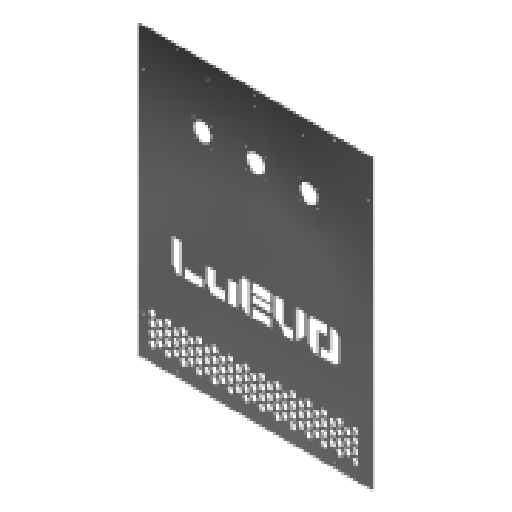
# Autodesk Inventor part: Extruder Side Panel
Saved by Autodesk Inventor 2023.2 (Build 272271000, 271)
## iProperties
Created: 2023-02-06
Part Number: Extruder Side Panel
Material: Aluminum 6061
Document SubType Name: Modeling
Designer: remop
Density: 2.7 g/cm^3
Appearance: Aluminum - Flat
Author: remop
Autodesk Inventor part; units mm, degrees
(part 1 of 2)
ref_plane "YZ Plane" through (0, 0, 0) normal (1, 0, 0) x (0, 1, 0)
ref_plane "XZ Plane" through (0, 0, 0) normal (0, 1, 0) x (-1, 0, 0)
ref_plane "XY Plane" through (0, 0, 0) normal (0, 0, 1) x (1, 0, 0)
sketch "Sketch1" plane through (0, 0, 0) normal (0, 0, 1) x (1, 0, 0)
  line L0 (-15, -15) -> (-15, 0) projected
  line L1 (0, -15) -> (-15, -15) projected
  line L2 (0, 0) -> (0, -15) projected
  line L3 (-15, 0) -> (0, 0) projected
  line L4 (360, 0) -> (360, -15) projected
  line L5 (360, -15) -> (375, -15) projected
  line L6 (375, -15) -> (375, 0) projected
  line L7 (375, 0) -> (360, 0) projected
  line L8 (360, -465) -> (360, -480) projected
  line L9 (360, -480) -> (375, -480) projected
  line L10 (375, -465) -> (375, -480) projected
  line L11 (360, -465) -> (375, -465) projected
  line L12 (0, -480) -> (0, -465) projected
  line L13 (0, -465) -> (-15, -465) projected
  line L14 (-15, -465) -> (-15, -480) projected
  line L15 (-15, -480) -> (0, -480) projected
  line L16 (375, -465) -> (375, -15)
  line L17 (360, 0) -> (0, 0)
  line L18 (-15, -15) -> (-15, -465)
  line L19 (0, -480) -> (360, -480)
  circle A0 centre (-7.5, -65) radius 1.75
  circle A1 centre (-7.5, -415) radius 1.75
  circle A2 centre (367.5, -65) radius 1.75
  circle A3 centre (367.5, -415) radius 1.75
  circle A4 centre (50, -7.5) radius 1.75
  circle A5 centre (310, -7.5) radius 1.75
  circle A6 centre (310, -472.5) radius 1.75
  circle A7 centre (50, -472.5) radius 1.75
  circle A8 centre (180, -7.5) radius 1.75
  circle A9 centre (180, -25) radius 1.75
  circle A10 centre (100, -25) radius 1.75
  circle A11 centre (260, -25) radius 1.75
  point P0 (367.5, -15)
  point P1 (367.5, -465)
  point P2 (-7.5, -465)
  point P3 (-7.5, -15)
  point P4 (0, -472.5)
  point P5 (360, -472.5)
  point P6 (0, -7.5)
  point P7 (360, -7.5)
  point P8 (180, -480)
  dimension "d0" = 50
  dimension "d1" = 3.5
  dimension "d2" = 50
  dimension "d3" = 50
  dimension "d4" = 50
  dimension "d5" = 50
  dimension "d6" = 50
  dimension "d68" = 17.5
  dimension "d69" = 80
  dimension "d70" = 80
  constraints: 12 centre point, 11 equal radius, 9 horizontal alignment, 9 midpoint, 8 end point, 6 vertical alignment, 2 perpendicular, 1 parallel, 1 vertical
  measures "d0" distance from line of A0.centre L1
  measures "d1" diameter of A2
  measures "d2" distance from line of L13 A1.centre
  measures "d3" distance from line of L12 A7.centre
  measures "d4" distance from line of A6.centre L8
  measures "d5" distance from line of L4 A5.centre
  measures "d6" distance from line of L2 A4.centre
  measures "d68" distance of A9.centre A8.centre
  measures "d69" distance of A9.centre A10.centre
  measures "d70" distance of A9.centre A11.centre
extrude "Extrusion1" add sketch "Sketch1" along normal blind 2
sketch "Sketch2" plane through (0, 0, 2) normal (0, 0, 1) x (1, 0, 0)
  line L0 (-15, -480) -> (375, -480) projected
  line L1 (375, -480) -> (375, 0) projected
  line L2 (375, 0) -> (-15, 0) projected
  line L3 (-15, 0) -> (-15, -480) projected
  circle A0 centre (50, -472.5) radius 1.75 projected
  circle A1 centre (310, -472.5) radius 1.75 projected
  circle A2 centre (310, -7.5) radius 1.75 projected
  circle A3 centre (50, -7.5) radius 1.75 projected
  circle A4 centre (367.5, -415) radius 1.75 projected
  circle A5 centre (367.5, -65) radius 1.75 projected
  circle A6 centre (-7.5, -415) radius 1.75 projected
  circle A7 centre (-7.5, -65) radius 1.75 projected
  point P0 (0, 0)
  point P1 (283.5, -90)
  point P2 (252.5, -90)
  point P3 (283.5, -121)
  point P4 (252.5, -121)
  point P5 (195.5, -90)
  point P6 (164.5, -90)
  point P7 (164.5, -121)
  point P8 (195.5, -121)
  point P9 (107.5, -90)
  point P10 (76.5, -90)
  point P11 (76.5, -121)
  point P12 (107.5, -121)
  point P13 (180, 0)
  dimension "d11" = 31
  dimension "d14" = 31
  dimension "d19" = 88
  dimension "d24" = 90
  dimension "d25" = 15.5
  constraints: 2 horizontal, 1 midpoint, 1 vertical, 11 other
  measures "d11" distance of point (283.5, -90) point (252.5, -90)
  measures "d14" distance of point (283.5, -90) point (283.5, -121)
  measures "d19" distance of point (283.5, -90) point (195.5, -90)
  measures "d24" distance from line of L2 point (76.5, -90)
  measures "d25" horizontal distance of point (180, 0) point (195.5, -90)
hole "Extruder Mount" at (283.5, -90, 2) at (252.5, -90, 2) at (283.5, -121, 2) at (252.5, -121, 2) at (195.5, -90, 2) at (164.5, -90, 2) at (164.5, -121, 2) at (195.5, -121, 2) at (107.5, -90, 2) at (76.5, -90, 2) at (76.5, -121, 2) at (107.5, -121, 2) direction (0, 0, -1) diameter 3.5 end through all
sketch "Sketch3" plane through (0, 0, 2) normal (0, 0, 1) x (1, 0, 0)
  circle A0 centre (92, -105.5) radius 15
  circle A1 centre (180, -105.5) radius 15
  circle A2 centre (268, -105.5) radius 15
  line L0 (375, 0) -> (-15, 0) projected
  point P0 (0, 0)
  point P1 (180, 0)
  dimension "d33" = 105.5
  dimension "d34" = 30
  dimension "d35" = 88
  dimension "d36" = 88
  constraints: 3 centre point, 2 equal radius, 2 horizontal alignment, 1 midpoint, 1 vertical alignment
  measures "d33" distance from line of L0 A1.centre
  measures "d34" diameter of A1
  measures "d35" distance of A1.centre A2.centre
  measures "d36" distance of A1.centre A0.centre
extrude "Extrusion2" cut sketch "Sketch3" against normal through all
sketch "Sketch4" plane through (0, 0, 2) normal (0, 0, 1) x (1, 0, 0)
  circle A0 centre (268, -105.5) radius 15 projected
  circle A1 centre (180, -105.5) radius 15 projected
  circle A2 centre (92, -105.5) radius 15 projected
  circle A3 centre (76.5, -121) radius 1.75 projected
  circle A4 centre (107.5, -90) radius 1.75 projected
  circle A5 centre (164.5, -121) radius 1.75 projected
  circle A6 centre (195.5, -90) radius 1.75 projected
  circle A7 centre (283.5, -121) radius 1.75 projected
  circle A8 centre (283.5, -90) radius 1.75 projected
  circle A9 centre (252.5, -90) radius 1.75 projected
  circle A10 centre (252.5, -121) radius 1.75 projected
  circle A11 centre (164.5, -90) radius 1.75 projected
  circle A12 centre (195.5, -121) radius 1.75 projected
  circle A13 centre (76.5, -90) radius 1.75 projected
  circle A14 centre (107.5, -121) radius 1.75 projected
  line L0 (-15, -480) -> (375, -480) projected
  line L1 (375, -480) -> (375, 0) projected
  line L2 (375, 0) -> (-15, 0) projected
  line L3 (-15, 0) -> (-15, -480) projected
  circle A15 centre (50, -472.5) radius 1.75 projected
  circle A16 centre (310, -472.5) radius 1.75 projected
  circle A17 centre (310, -7.5) radius 1.75 projected
  circle A18 centre (50, -7.5) radius 1.75 projected
  circle A19 centre (367.5, -415) radius 1.75 projected
  circle A20 centre (367.5, -65) radius 1.75 projected
  circle A21 centre (-7.5, -415) radius 1.75 projected
  circle A22 centre (-7.5, -65) radius 1.75 projected
  line L4 (10.9983, -458) -> (5.2247, -458)
  line L5 (5.2247, -458) -> (2.338, -453)
  line L6 (2.338, -453) -> (5.2247, -448)
  line L7 (5.2247, -448) -> (10.9983, -448)
  line L8 (10.9983, -448) -> (13.885, -453)
  line L9 (13.885, -453) -> (10.9983, -458)
  line L10 (18.2151, -450.5) -> (15.3284, -445.5)
  line L11 (15.3284, -445.5) -> (18.2151, -440.5)
  line L12 (18.2151, -440.5) -> (23.9886, -440.5)
  line L13 (23.9886, -440.5) -> (26.8754, -445.5)
  line L14 (26.8754, -445.5) -> (23.9886, -450.5)
  line L15 (23.9886, -450.5) -> (18.2151, -450.5)
  line L16 (10.9983, -443) -> (5.2247, -443)
  line L17 (5.2247, -443) -> (2.338, -438)
  line L18 (2.338, -438) -> (5.2247, -433)
  line L19 (5.2247, -433) -> (10.9983, -433)
  line L20 (10.9983, -433) -> (13.885, -438)
  line L21 (13.885, -438) -> (10.9983, -443)
  line L22 (5.2247, -418) -> (10.9983, -418)
  line L23 (2.338, -423) -> (5.2247, -418)
  line L24 (10.9983, -418) -> (13.885, -423)
  line L25 (18.2151, -425.5) -> (23.9886, -425.5)
  line L26 (5.2247, -428) -> (2.338, -423)
  line L27 (10.9983, -428) -> (5.2247, -428)
  line L28 (13.885, -423) -> (10.9983, -428)
  line L29 (15.3284, -430.5) -> (18.2151, -425.5)
  line L30 (23.9886, -425.5) -> (26.8754, -430.5)
  line L31 (18.2151, -435.5) -> (15.3284, -430.5)
  line L32 (23.9886, -435.5) -> (18.2151, -435.5)
  line L33 (26.8754, -430.5) -> (23.9886, -435.5)
  line L34 (5.2247, -403) -> (10.9983, -403)
  line L35 (2.338, -408) -> (5.2247, -403)
  line L36 (10.9983, -403) -> (13.885, -408)
  line L37 (18.2151, -410.5) -> (23.9886, -410.5)
  line L38 (5.2247, -413) -> (2.338, -408)
  line L39 (10.9983, -413) -> (5.2247, -413)
  line L40 (13.885, -408) -> (10.9983, -413)
  line L41 (15.3284, -415.5) -> (18.2151, -410.5)
  line L42 (23.9886, -410.5) -> (26.8754, -415.5)
  line L43 (18.2151, -420.5) -> (15.3284, -415.5)
  line L44 (23.9886, -420.5) -> (18.2151, -420.5)
  line L45 (26.8754, -415.5) -> (23.9886, -420.5)
  line L46 (36.9983, -403) -> (39.885, -408)
  line L47 (31.2247, -403) -> (36.9983, -403)
  line L48 (39.885, -408) -> (36.9983, -413)
  line L49 (28.338, -408) -> (31.2247, -403)
  line L50 (31.2247, -413) -> (28.338, -408)
  line L51 (36.9983, -413) -> (31.2247, -413)
  line L52 (44.2151, -450.5) -> (41.3284, -445.5)
  line L53 (41.3284, -445.5) -> (44.2151, -440.5)
  line L54 (44.2151, -440.5) -> (49.9886, -440.5)
  line L55 (49.9886, -440.5) -> (52.8754, -445.5)
  line L56 (49.9886, -450.5) -> (44.2151, -450.5)
  line L57 (52.8754, -445.5) -> (49.9886, -450.5)
  line L58 (36.9983, -458) -> (31.2247, -458)
  line L59 (36.9983, -448) -> (39.885, -453)
  line L60 (39.885, -438) -> (36.9983, -443)
  line L61 (39.885, -453) -> (36.9983, -458)
  line L62 (31.2247, -448) -> (36.9983, -448)
  line L63 (31.2247, -458) -> (28.338, -453)
  line L64 (28.338, -453) -> (31.2247, -448)
  line L65 (36.9983, -433) -> (39.885, -438)
  line L66 (36.9983, -443) -> (31.2247, -443)
  line L67 (31.2247, -443) -> (28.338, -438)
  line L68 (31.2247, -433) -> (36.9983, -433)
  line L69 (28.338, -438) -> (31.2247, -433)
  line L70 (36.9983, -428) -> (31.2247, -428)
  line L71 (39.885, -423) -> (36.9983, -428)
  line L72 (31.2247, -428) -> (28.338, -423)
  line L73 (36.9983, -418) -> (39.885, -423)
  line L74 (31.2247, -418) -> (36.9983, -418)
  line L75 (28.338, -423) -> (31.2247, -418)
  line L76 (41.3284, -430.5) -> (44.2151, -425.5)
  line L77 (44.2151, -435.5) -> (41.3284, -430.5)
  line L78 (49.9886, -435.5) -> (44.2151, -435.5)
  line L79 (52.8754, -430.5) -> (49.9886, -435.5)
  line L80 (49.9886, -425.5) -> (52.8754, -430.5)
  line L81 (44.2151, -425.5) -> (49.9886, -425.5)
  line L82 (44.2151, -420.5) -> (41.3284, -415.5)
  line L83 (41.3284, -415.5) -> (44.2151, -410.5)
  line L84 (49.9886, -420.5) -> (44.2151, -420.5)
  line L85 (44.2151, -410.5) -> (49.9886, -410.5)
  line L86 (52.8754, -415.5) -> (49.9886, -420.5)
  line L87 (49.9886, -410.5) -> (52.8754, -415.5)
  line L88 (62.9983, -403) -> (65.885, -408)
  line L89 (57.2247, -403) -> (62.9983, -403)
  line L90 (65.885, -408) -> (62.9983, -413)
  line L91 (54.338, -408) -> (57.2247, -403)
  line L92 (57.2247, -413) -> (54.338, -408)
  line L93 (62.9983, -413) -> (57.2247, -413)
  line L94 (70.2151, -450.5) -> (67.3284, -445.5)
  line L95 (67.3284, -445.5) -> (70.2151, -440.5)
  line L96 (70.2151, -440.5) -> (75.9886, -440.5)
  line L97 (75.9886, -440.5) -> (78.8754, -445.5)
  line L98 (75.9886, -450.5) -> (70.2151, -450.5)
  line L99 (78.8754, -445.5) -> (75.9886, -450.5)
  line L100 (62.9983, -458) -> (57.2247, -458)
  line L101 (62.9983, -448) -> (65.885, -453)
  line L102 (65.885, -438) -> (62.9983, -443)
  line L103 (65.885, -453) -> (62.9983, -458)
  line L104 (57.2247, -448) -> (62.9983, -448)
  line L105 (57.2247, -458) -> (54.338, -453)
  line L106 (54.338, -453) -> (57.2247, -448)
  line L107 (62.9983, -433) -> (65.885, -438)
  line L108 (62.9983, -443) -> (57.2247, -443)
  line L109 (57.2247, -443) -> (54.338, -438)
  line L110 (57.2247, -433) -> (62.9983, -433)
  line L111 (54.338, -438) -> (57.2247, -433)
  line L112 (62.9983, -428) -> (57.2247, -428)
  line L113 (65.885, -423) -> (62.9983, -428)
  line L114 (57.2247, -428) -> (54.338, -423)
  line L115 (62.9983, -418) -> (65.885, -423)
  line L116 (57.2247, -418) -> (62.9983, -418)
  line L117 (54.338, -423) -> (57.2247, -418)
  line L118 (67.3284, -430.5) -> (70.2151, -425.5)
  line L119 (70.2151, -435.5) -> (67.3284, -430.5)
  line L120 (75.9886, -435.5) -> (70.2151, -435.5)
  line L121 (78.8754, -430.5) -> (75.9886, -435.5)
  line L122 (75.9886, -425.5) -> (78.8754, -430.5)
  line L123 (70.2151, -425.5) -> (75.9886, -425.5)
  line L124 (70.2151, -420.5) -> (67.3284, -415.5)
  line L125 (67.3284, -415.5) -> (70.2151, -410.5)
  line L126 (75.9886, -420.5) -> (70.2151, -420.5)
  line L127 (70.2151, -410.5) -> (75.9886, -410.5)
  line L128 (78.8754, -415.5) -> (75.9886, -420.5)
  line L129 (75.9886, -410.5) -> (78.8754, -415.5)
  line L130 (88.9983, -403) -> (91.885, -408)
  line L131 (83.2247, -403) -> (88.9983, -403)
  line L132 (91.885, -408) -> (88.9983, -413)
  line L133 (80.338, -408) -> (83.2247, -403)
  line L134 (83.2247, -413) -> (80.338, -408)
  line L135 (88.9983, -413) -> (83.2247, -413)
  line L136 (96.2151, -450.5) -> (93.3284, -445.5)
  line L137 (93.3284, -445.5) -> (96.2151, -440.5)
  line L138 (96.2151, -440.5) -> (101.9886, -440.5)
  line L139 (101.9886, -440.5) -> (104.8754, -445.5)
  line L140 (101.9886, -450.5) -> (96.2151, -450.5)
  line L141 (104.8754, -445.5) -> (101.9886, -450.5)
  line L142 (88.9983, -458) -> (83.2247, -458)
  line L143 (88.9983, -448) -> (91.885, -453)
  line L144 (91.885, -438) -> (88.9983, -443)
  line L145 (91.885, -453) -> (88.9983, -458)
  line L146 (83.2247, -448) -> (88.9983, -448)
  line L147 (83.2247, -458) -> (80.338, -453)
  line L148 (80.338, -453) -> (83.2247, -448)
  line L149 (88.9983, -433) -> (91.885, -438)
  line L150 (88.9983, -443) -> (83.2247, -443)
  line L151 (83.2247, -443) -> (80.338, -438)
  line L152 (83.2247, -433) -> (88.9983, -433)
  line L153 (80.338, -438) -> (83.2247, -433)
  line L154 (88.9983, -428) -> (83.2247, -428)
  line L155 (91.885, -423) -> (88.9983, -428)
  line L156 (83.2247, -428) -> (80.338, -423)
  line L157 (88.9983, -418) -> (91.885, -423)
  line L158 (83.2247, -418) -> (88.9983, -418)
  line L159 (80.338, -423) -> (83.2247, -418)
  line L160 (93.3284, -430.5) -> (96.2151, -425.5)
  line L161 (96.2151, -435.5) -> (93.3284, -430.5)
  line L162 (101.9886, -435.5) -> (96.2151, -435.5)
  line L163 (104.8754, -430.5) -> (101.9886, -435.5)
  line L164 (101.9886, -425.5) -> (104.8754, -430.5)
  line L165 (96.2151, -425.5) -> (101.9886, -425.5)
  line L166 (96.2151, -420.5) -> (93.3284, -415.5)
  line L167 (93.3284, -415.5) -> (96.2151, -410.5)
  line L168 (101.9886, -420.5) -> (96.2151, -420.5)
  line L169 (96.2151, -410.5) -> (101.9886, -410.5)
  line L170 (104.8754, -415.5) -> (101.9886, -420.5)
  line L171 (101.9886, -410.5) -> (104.8754, -415.5)
  line L172 (114.9983, -403) -> (117.885, -408)
  line L173 (109.2247, -403) -> (114.9983, -403)
  line L174 (117.885, -408) -> (114.9983, -413)
  line L175 (106.338, -408) -> (109.2247, -403)
  line L176 (109.2247, -413) -> (106.338, -408)
  line L177 (114.9983, -413) -> (109.2247, -413)
  line L178 (122.2151, -450.5) -> (119.3284, -445.5)
  line L179 (119.3284, -445.5) -> (122.2151, -440.5)
  line L180 (122.2151, -440.5) -> (127.9886, -440.5)
  line L181 (127.9886, -440.5) -> (130.8754, -445.5)
  line L182 (127.9886, -450.5) -> (122.2151, -450.5)
  line L183 (130.8754, -445.5) -> (127.9886, -450.5)
  line L184 (114.9983, -458) -> (109.2247, -458)
  line L185 (114.9983, -448) -> (117.885, -453)
  line L186 (117.885, -438) -> (114.9983, -443)
  line L187 (117.885, -453) -> (114.9983, -458)
  line L188 (109.2247, -448) -> (114.9983, -448)
  line L189 (109.2247, -458) -> (106.338, -453)
  line L190 (106.338, -453) -> (109.2247, -448)
  line L191 (114.9983, -433) -> (117.885, -438)
  line L192 (114.9983, -443) -> (109.2247, -443)
  line L193 (109.2247, -443) -> (106.338, -438)
  line L194 (109.2247, -433) -> (114.9983, -433)
  line L195 (106.338, -438) -> (109.2247, -433)
  line L196 (114.9983, -428) -> (109.2247, -428)
  line L197 (117.885, -423) -> (114.9983, -428)
  line L198 (109.2247, -428) -> (106.338, -423)
  line L199 (114.9983, -418) -> (117.885, -423)
  line L200 (109.2247, -418) -> (114.9983, -418)
  line L201 (106.338, -423) -> (109.2247, -418)
  line L202 (119.3284, -430.5) -> (122.2151, -425.5)
  line L203 (122.2151, -435.5) -> (119.3284, -430.5)
  line L204 (127.9886, -435.5) -> (122.2151, -435.5)
  line L205 (130.8754, -430.5) -> (127.9886, -435.5)
  line L206 (127.9886, -425.5) -> (130.8754, -430.5)
  line L207 (122.2151, -425.5) -> (127.9886, -425.5)
  line L208 (122.2151, -420.5) -> (119.3284, -415.5)
  line L209 (119.3284, -415.5) -> (122.2151, -410.5)
  line L210 (127.9886, -420.5) -> (122.2151, -420.5)
  line L211 (122.2151, -410.5) -> (127.9886, -410.5)
  line L212 (130.8754, -415.5) -> (127.9886, -420.5)
  line L213 (127.9886, -410.5) -> (130.8754, -415.5)
  line L214 (140.9983, -403) -> (143.885, -408)
  line L215 (135.2247, -403) -> (140.9983, -403)
  line L216 (143.885, -408) -> (140.9983, -413)
  line L217 (132.338, -408) -> (135.2247, -403)
  line L218 (135.2247, -413) -> (132.338, -408)
  line L219 (140.9983, -413) -> (135.2247, -413)
  line L220 (148.2151, -450.5) -> (145.3284, -445.5)
  line L221 (145.3284, -445.5) -> (148.2151, -440.5)
  line L222 (148.2151, -440.5) -> (153.9886, -440.5)
  line L223 (153.9886, -440.5) -> (156.8754, -445.5)
  line L224 (153.9886, -450.5) -> (148.2151, -450.5)
  line L225 (156.8754, -445.5) -> (153.9886, -450.5)
  line L226 (140.9983, -458) -> (135.2247, -458)
  line L227 (140.9983, -448) -> (143.885, -453)
  line L228 (143.885, -438) -> (140.9983, -443)
  line L229 (143.885, -453) -> (140.9983, -458)
  line L230 (135.2247, -448) -> (140.9983, -448)
  line L231 (135.2247, -458) -> (132.338, -453)
  line L232 (132.338, -453) -> (135.2247, -448)
  line L233 (140.9983, -433) -> (143.885, -438)
  line L234 (140.9983, -443) -> (135.2247, -443)
  line L235 (135.2247, -443) -> (132.338, -438)
  line L236 (135.2247, -433) -> (140.9983, -433)
  line L237 (132.338, -438) -> (135.2247, -433)
  line L238 (140.9983, -428) -> (135.2247, -428)
  line L239 (143.885, -423) -> (140.9983, -428)
  line L240 (135.2247, -428) -> (132.338, -423)
  line L241 (140.9983, -418) -> (143.885, -423)
  line L242 (135.2247, -418) -> (140.9983, -418)
  line L243 (132.338, -423) -> (135.2247, -418)
  line L244 (145.3284, -430.5) -> (148.2151, -425.5)
  line L245 (148.2151, -435.5) -> (145.3284, -430.5)
  line L246 (153.9886, -435.5) -> (148.2151, -435.5)
  line L247 (156.8754, -430.5) -> (153.9886, -435.5)
  line L248 (153.9886, -425.5) -> (156.8754, -430.5)
  line L249 (148.2151, -425.5) -> (153.9886, -425.5)
  line L250 (148.2151, -420.5) -> (145.3284, -415.5)
  line L251 (145.3284, -415.5) -> (148.2151, -410.5)
  line L252 (153.9886, -420.5) -> (148.2151, -420.5)
  line L253 (148.2151, -410.5) -> (153.9886, -410.5)
  line L254 (156.8754, -415.5) -> (153.9886, -420.5)
  line L255 (153.9886, -410.5) -> (156.8754, -415.5)
  line L256 (166.9983, -403) -> (169.885, -408)
  line L257 (161.2247, -403) -> (166.9983, -403)
  line L258 (169.885, -408) -> (166.9983, -413)
  line L259 (158.338, -408) -> (161.2247, -403)
  line L260 (161.2247, -413) -> (158.338, -408)
  line L261 (166.9983, -413) -> (161.2247, -413)
  line L262 (174.2151, -450.5) -> (171.3284, -445.5)
  line L263 (171.3284, -445.5) -> (174.2151, -440.5)
  line L264 (174.2151, -440.5) -> (179.9886, -440.5)
  line L265 (179.9886, -440.5) -> (182.8754, -445.5)
  line L266 (179.9886, -450.5) -> (174.2151, -450.5)
  line L267 (182.8754, -445.5) -> (179.9886, -450.5)
  line L268 (166.9983, -458) -> (161.2247, -458)
  line L269 (166.9983, -448) -> (169.885, -453)
  line L270 (169.885, -438) -> (166.9983, -443)
  line L271 (169.885, -453) -> (166.9983, -458)
  line L272 (161.2247, -448) -> (166.9983, -448)
  line L273 (161.2247, -458) -> (158.338, -453)
  line L274 (158.338, -453) -> (161.2247, -448)
  line L275 (166.9983, -433) -> (169.885, -438)
  line L276 (166.9983, -443) -> (161.2247, -443)
  line L277 (161.2247, -443) -> (158.338, -438)
  line L278 (161.2247, -433) -> (166.9983, -433)
  line L279 (158.338, -438) -> (161.2247, -433)
  line L280 (166.9983, -428) -> (161.2247, -428)
  line L281 (169.885, -423) -> (166.9983, -428)
  line L282 (161.2247, -428) -> (158.338, -423)
  line L283 (166.9983, -418) -> (169.885, -423)
  line L284 (161.2247, -418) -> (166.9983, -418)
  line L285 (158.338, -423) -> (161.2247, -418)
  line L286 (171.3284, -430.5) -> (174.2151, -425.5)
  line L287 (174.2151, -435.5) -> (171.3284, -430.5)
  line L288 (179.9886, -435.5) -> (174.2151, -435.5)
  line L289 (182.8754, -430.5) -> (179.9886, -435.5)
  line L290 (179.9886, -425.5) -> (182.8754, -430.5)
  line L291 (174.2151, -425.5) -> (179.9886, -425.5)
  line L292 (174.2151, -420.5) -> (171.3284, -415.5)
  line L293 (171.3284, -415.5) -> (174.2151, -410.5)
  line L294 (179.9886, -420.5) -> (174.2151, -420.5)
  line L295 (174.2151, -410.5) -> (179.9886, -410.5)
  line L296 (182.8754, -415.5) -> (179.9886, -420.5)
  line L297 (179.9886, -410.5) -> (182.8754, -415.5)
  line L298 (192.9983, -403) -> (195.885, -408)
  line L299 (187.2247, -403) -> (192.9983, -403)
  line L300 (195.885, -408) -> (192.9983, -413)
  line L301 (184.338, -408) -> (187.2247, -403)
  line L302 (187.2247, -413) -> (184.338, -408)
  line L303 (192.9983, -413) -> (187.2247, -413)
  line L304 (200.2151, -450.5) -> (197.3284, -445.5)
  line L305 (197.3284, -445.5) -> (200.2151, -440.5)
  line L306 (200.2151, -440.5) -> (205.9886, -440.5)
  line L307 (205.9886, -440.5) -> (208.8754, -445.5)
  line L308 (205.9886, -450.5) -> (200.2151, -450.5)
  line L309 (208.8754, -445.5) -> (205.9886, -450.5)
  line L310 (192.9983, -458) -> (187.2247, -458)
  line L311 (192.9983, -448) -> (195.885, -453)
  line L312 (195.885, -438) -> (192.9983, -443)
  line L313 (195.885, -453) -> (192.9983, -458)
  line L314 (187.2247, -448) -> (192.9983, -448)
  line L315 (187.2247, -458) -> (184.338, -453)
  line L316 (184.338, -453) -> (187.2247, -448)
  line L317 (192.9983, -433) -> (195.885, -438)
  line L318 (192.9983, -443) -> (187.2247, -443)
  line L319 (187.2247, -443) -> (184.338, -438)
  line L320 (187.2247, -433) -> (192.9983, -433)
  line L321 (184.338, -438) -> (187.2247, -433)
  line L322 (192.9983, -428) -> (187.2247, -428)
  line L323 (195.885, -423) -> (192.9983, -428)
  line L324 (187.2247, -428) -> (184.338, -423)
  line L325 (192.9983, -418) -> (195.885, -423)
  line L326 (187.2247, -418) -> (192.9983, -418)
  line L327 (184.338, -423) -> (187.2247, -418)
  line L328 (197.3284, -430.5) -> (200.2151, -425.5)
  line L329 (200.2151, -435.5) -> (197.3284, -430.5)
  line L330 (205.9886, -435.5) -> (200.2151, -435.5)
  line L331 (208.8754, -430.5) -> (205.9886, -435.5)
  line L332 (205.9886, -425.5) -> (208.8754, -430.5)
  line L333 (200.2151, -425.5) -> (205.9886, -425.5)
  line L334 (200.2151, -420.5) -> (197.3284, -415.5)
  line L335 (197.3284, -415.5) -> (200.2151, -410.5)
  line L336 (205.9886, -420.5) -> (200.2151, -420.5)
  line L337 (200.2151, -410.5) -> (205.9886, -410.5)
  line L338 (208.8754, -415.5) -> (205.9886, -420.5)
  line L339 (205.9886, -410.5) -> (208.8754, -415.5)
  line L340 (218.9983, -403) -> (221.885, -408)
  line L341 (213.2247, -403) -> (218.9983, -403)
  line L342 (221.885, -408) -> (218.9983, -413)
  line L343 (210.338, -408) -> (213.2247, -403)
  line L344 (213.2247, -413) -> (210.338, -408)
  line L345 (218.9983, -413) -> (213.2247, -413)
  line L346 (226.2151, -450.5) -> (223.3284, -445.5)
  line L347 (223.3284, -445.5) -> (226.2151, -440.5)
  line L348 (226.2151, -440.5) -> (231.9886, -440.5)
  line L349 (231.9886, -440.5) -> (234.8754, -445.5)
  line L350 (231.9886, -450.5) -> (226.2151, -450.5)
  line L351 (234.8754, -445.5) -> (231.9886, -450.5)
  line L352 (218.9983, -458) -> (213.2247, -458)
  line L353 (218.9983, -448) -> (221.885, -453)
  line L354 (221.885, -438) -> (218.9983, -443)
  line L355 (221.885, -453) -> (218.9983, -458)
  line L356 (213.2247, -448) -> (218.9983, -448)
  line L357 (213.2247, -458) -> (210.338, -453)
  line L358 (210.338, -453) -> (213.2247, -448)
  line L359 (218.9983, -433) -> (221.885, -438)
  line L360 (218.9983, -443) -> (213.2247, -443)
  line L361 (213.2247, -443) -> (210.338, -438)
  line L362 (213.2247, -433) -> (218.9983, -433)
  line L363 (210.338, -438) -> (213.2247, -433)
  line L364 (218.9983, -428) -> (213.2247, -428)
  line L365 (221.885, -423) -> (218.9983, -428)
  line L366 (213.2247, -428) -> (210.338, -423)
  line L367 (218.9983, -418) -> (221.885, -423)
  line L368 (213.2247, -418) -> (218.9983, -418)
  line L369 (210.338, -423) -> (213.2247, -418)
  line L370 (223.3284, -430.5) -> (226.2151, -425.5)
  line L371 (226.2151, -435.5) -> (223.3284, -430.5)
  line L372 (231.9886, -435.5) -> (226.2151, -435.5)
  line L373 (234.8754, -430.5) -> (231.9886, -435.5)
  line L374 (231.9886, -425.5) -> (234.8754, -430.5)
  line L375 (226.2151, -425.5) -> (231.9886, -425.5)
  line L376 (226.2151, -420.5) -> (223.3284, -415.5)
  line L377 (223.3284, -415.5) -> (226.2151, -410.5)
  line L378 (231.9886, -420.5) -> (226.2151, -420.5)
  line L379 (226.2151, -410.5) -> (231.9886, -410.5)
  line L380 (234.8754, -415.5) -> (231.9886, -420.5)
  line L381 (231.9886, -410.5) -> (234.8754, -415.5)
  line L382 (244.9983, -403) -> (247.885, -408)
  line L383 (239.2247, -403) -> (244.9983, -403)
  line L384 (247.885, -408) -> (244.9983, -413)
  line L385 (236.338, -408) -> (239.2247, -403)
  line L386 (239.2247, -413) -> (236.338, -408)
  line L387 (244.9983, -413) -> (239.2247, -413)
  line L388 (252.2151, -450.5) -> (249.3284, -445.5)
  line L389 (249.3284, -445.5) -> (252.2151, -440.5)
  line L390 (252.2151, -440.5) -> (257.9886, -440.5)
  line L391 (257.9886, -440.5) -> (260.8754, -445.5)
  line L392 (257.9886, -450.5) -> (252.2151, -450.5)
  line L393 (260.8754, -445.5) -> (257.9886, -450.5)
  line L394 (244.9983, -458) -> (239.2247, -458)
  line L395 (244.9983, -448) -> (247.885, -453)
  line L396 (247.885, -438) -> (244.9983, -443)
  line L397 (247.885, -453) -> (244.9983, -458)
  line L398 (239.2247, -448) -> (244.9983, -448)
  line L399 (239.2247, -458) -> (236.338, -453)
  line L400 (236.338, -453) -> (239.2247, -448)
  line L401 (244.9983, -433) -> (247.885, -438)
  line L402 (244.9983, -443) -> (239.2247, -443)
  line L403 (239.2247, -443) -> (236.338, -438)
  line L404 (239.2247, -433) -> (244.9983, -433)
  line L405 (236.338, -438) -> (239.2247, -433)
  line L406 (244.9983, -428) -> (239.2247, -428)
  line L407 (247.885, -423) -> (244.9983, -428)
  line L408 (239.2247, -428) -> (236.338, -423)
  line L409 (244.9983, -418) -> (247.885, -423)
  line L410 (239.2247, -418) -> (244.9983, -418)
  line L411 (236.338, -423) -> (239.2247, -418)
  line L412 (249.3284, -430.5) -> (252.2151, -425.5)
  line L413 (252.2151, -435.5) -> (249.3284, -430.5)
  line L414 (257.9886, -435.5) -> (252.2151, -435.5)
  line L415 (260.8754, -430.5) -> (257.9886, -435.5)
  line L416 (257.9886, -425.5) -> (260.8754, -430.5)
  line L417 (252.2151, -425.5) -> (257.9886, -425.5)
  line L418 (252.2151, -420.5) -> (249.3284, -415.5)
  line L419 (249.3284, -415.5) -> (252.2151, -410.5)
  line L420 (257.9886, -420.5) -> (252.2151, -420.5)
  line L421 (252.2151, -410.5) -> (257.9886, -410.5)
  line L422 (260.8754, -415.5) -> (257.9886, -420.5)
  line L423 (257.9886, -410.5) -> (260.8754, -415.5)
  line L424 (270.9983, -403) -> (273.885, -408)
  line L425 (265.2247, -403) -> (270.9983, -403)
  line L426 (273.885, -408) -> (270.9983, -413)
  line L427 (262.338, -408) -> (265.2247, -403)
  line L428 (265.2247, -413) -> (262.338, -408)
  line L429 (270.9983, -413) -> (265.2247, -413)
  line L430 (278.2151, -450.5) -> (275.3284, -445.5)
  line L431 (275.3284, -445.5) -> (278.2151, -440.5)
  line L432 (278.2151, -440.5) -> (283.9886, -440.5)
  line L433 (283.9886, -440.5) -> (286.8754, -445.5)
  line L434 (283.9886, -450.5) -> (278.2151, -450.5)
  line L435 (286.8754, -445.5) -> (283.9886, -450.5)
  line L436 (270.9983, -458) -> (265.2247, -458)
  line L437 (270.9983, -448) -> (273.885, -453)
  line L438 (273.885, -438) -> (270.9983, -443)
  line L439 (273.885, -453) -> (270.9983, -458)
  line L440 (265.2247, -448) -> (270.9983, -448)
  line L441 (265.2247, -458) -> (262.338, -453)
  line L442 (262.338, -453) -> (265.2247, -448)
  line L443 (270.9983, -433) -> (273.885, -438)
  line L444 (270.9983, -443) -> (265.2247, -443)
  line L445 (265.2247, -443) -> (262.338, -438)
  line L446 (265.2247, -433) -> (270.9983, -433)
  line L447 (262.338, -438) -> (265.2247, -433)
  line L448 (270.9983, -428) -> (265.2247, -428)
  line L449 (273.885, -423) -> (270.9983, -428)
  line L450 (265.2247, -428) -> (262.338, -423)
  line L451 (270.9983, -418) -> (273.885, -423)
  line L452 (265.2247, -418) -> (270.9983, -418)
  line L453 (262.338, -423) -> (265.2247, -418)
  line L454 (275.3284, -430.5) -> (278.2151, -425.5)
  line L455 (278.2151, -435.5) -> (275.3284, -430.5)
  line L456 (283.9886, -435.5) -> (278.2151, -435.5)
  line L457 (286.8754, -430.5) -> (283.9886, -435.5)
  line L458 (283.9886, -425.5) -> (286.8754, -430.5)
  line L459 (278.2151, -425.5) -> (283.9886, -425.5)
  line L460 (278.2151, -420.5) -> (275.3284, -415.5)
  line L461 (275.3284, -415.5) -> (278.2151, -410.5)
  line L462 (283.9886, -420.5) -> (278.2151, -420.5)
  line L463 (278.2151, -410.5) -> (283.9886, -410.5)
  line L464 (286.8754, -415.5) -> (283.9886, -420.5)
  line L465 (283.9886, -410.5) -> (286.8754, -415.5)
  line L466 (296.9983, -403) -> (299.885, -408)
  line L467 (291.2247, -403) -> (296.9983, -403)
  line L468 (299.885, -408) -> (296.9983, -413)
  line L469 (288.338, -408) -> (291.2247, -403)
  line L470 (291.2247, -413) -> (288.338, -408)
  line L471 (296.9983, -413) -> (291.2247, -413)
  line L472 (304.2151, -450.5) -> (301.3284, -445.5)
  line L473 (301.3284, -445.5) -> (304.2151, -440.5)
  line L474 (304.2151, -440.5) -> (309.9886, -440.5)
  line L475 (309.9886, -440.5) -> (312.8754, -445.5)
  line L476 (309.9886, -450.5) -> (304.2151, -450.5)
  line L477 (312.8754, -445.5) -> (309.9886, -450.5)
  line L478 (296.9983, -458) -> (291.2247, -458)
  line L479 (296.9983, -448) -> (299.885, -453)
  line L480 (299.885, -438) -> (296.9983, -443)
  line L481 (299.885, -453) -> (296.9983, -458)
  line L482 (291.2247, -448) -> (296.9983, -448)
  line L483 (291.2247, -458) -> (288.338, -453)
  line L484 (288.338, -453) -> (291.2247, -448)
  line L485 (296.9983, -433) -> (299.885, -438)
  line L486 (296.9983, -443) -> (291.2247, -443)
  line L487 (291.2247, -443) -> (288.338, -438)
  line L488 (291.2247, -433) -> (296.9983, -433)
  line L489 (288.338, -438) -> (291.2247, -433)
  line L490 (296.9983, -428) -> (291.2247, -428)
  line L491 (299.885, -423) -> (296.9983, -428)
  line L492 (291.2247, -428) -> (288.338, -423)
  line L493 (296.9983, -418) -> (299.885, -423)
  line L494 (291.2247, -418) -> (296.9983, -418)
  line L495 (288.338, -423) -> (291.2247, -418)
  line L496 (301.3284, -430.5) -> (304.2151, -425.5)
  line L497 (304.2151, -435.5) -> (301.3284, -430.5)
  line L498 (309.9886, -435.5) -> (304.2151, -435.5)
  line L499 (312.8754, -430.5) -> (309.9886, -435.5)
  line L500 (309.9886, -425.5) -> (312.8754, -430.5)
  line L501 (304.2151, -425.5) -> (309.9886, -425.5)
  line L502 (304.2151, -420.5) -> (301.3284, -415.5)
  line L503 (301.3284, -415.5) -> (304.2151, -410.5)
  line L504 (309.9886, -420.5) -> (304.2151, -420.5)
  line L505 (304.2151, -410.5) -> (309.9886, -410.5)
  line L506 (312.8754, -415.5) -> (309.9886, -420.5)
  line L507 (309.9886, -410.5) -> (312.8754, -415.5)
  line L508 (322.9983, -403) -> (325.885, -408)
  line L509 (317.2247, -403) -> (322.9983, -403)
  line L510 (325.885, -408) -> (322.9983, -413)
  line L511 (314.338, -408) -> (317.2247, -403)
  line L512 (317.2247, -413) -> (314.338, -408)
  line L513 (322.9983, -413) -> (317.2247, -413)
  line L514 (330.2151, -450.5) -> (327.3284, -445.5)
  line L515 (327.3284, -445.5) -> (330.2151, -440.5)
  line L516 (330.2151, -440.5) -> (335.9886, -440.5)
  line L517 (335.9886, -440.5) -> (338.8754, -445.5)
  line L518 (335.9886, -450.5) -> (330.2151, -450.5)
  line L519 (338.8754, -445.5) -> (335.9886, -450.5)
  line L520 (322.9983, -458) -> (317.2247, -458)
  line L521 (322.9983, -448) -> (325.885, -453)
  line L522 (325.885, -438) -> (322.9983, -443)
  line L523 (325.885, -453) -> (322.9983, -458)
  line L524 (317.2247, -448) -> (322.9983, -448)
  line L525 (317.2247, -458) -> (314.338, -453)
  line L526 (314.338, -453) -> (317.2247, -448)
  line L527 (322.9983, -433) -> (325.885, -438)
  line L528 (322.9983, -443) -> (317.2247, -443)
  line L529 (317.2247, -443) -> (314.338, -438)
  line L530 (317.2247, -433) -> (322.9983, -433)
  line L531 (314.338, -438) -> (317.2247, -433)
  line L532 (322.9983, -428) -> (317.2247, -428)
  line L533 (325.885, -423) -> (322.9983, -428)
  line L534 (317.2247, -428) -> (314.338, -423)
  line L535 (322.9983, -418) -> (325.885, -423)
  line L536 (317.2247, -418) -> (322.9983, -418)
  line L537 (314.338, -423) -> (317.2247, -418)
  line L538 (327.3284, -430.5) -> (330.2151, -425.5)
  line L539 (330.2151, -435.5) -> (327.3284, -430.5)
  line L540 (335.9886, -435.5) -> (330.2151, -435.5)
  line L541 (338.8754, -430.5) -> (335.9886, -435.5)
  line L542 (335.9886, -425.5) -> (338.8754, -430.5)
  line L543 (330.2151, -425.5) -> (335.9886, -425.5)
  line L544 (330.2151, -420.5) -> (327.3284, -415.5)
  line L545 (327.3284, -415.5) -> (330.2151, -410.5)
  line L546 (335.9886, -420.5) -> (330.2151, -420.5)
  line L547 (330.2151, -410.5) -> (335.9886, -410.5)
  line L548 (338.8754, -415.5) -> (335.9886, -420.5)
  line L549 (335.9886, -410.5) -> (338.8754, -415.5)
  line L550 (348.9983, -403) -> (351.885, -408)
  line L551 (343.2247, -403) -> (348.9983, -403)
  line L552 (351.885, -408) -> (348.9983, -413)
  line L553 (340.338, -408) -> (343.2247, -403)
  line L554 (343.2247, -413) -> (340.338, -408)
  line L555 (348.9983, -413) -> (343.2247, -413)
  line L556 (356.2151, -450.5) -> (353.3284, -445.5)
  line L557 (353.3284, -445.5) -> (356.2151, -440.5)
  line L558 (356.2151, -440.5) -> (361.9886, -440.5)
  line L559 (361.9886, -440.5) -> (364.8754, -445.5)
  line L560 (361.9886, -450.5) -> (356.2151, -450.5)
  line L561 (364.8754, -445.5) -> (361.9886, -450.5)
  line L562 (348.9983, -458) -> (343.2247, -458)
  line L563 (348.9983, -448) -> (351.885, -453)
  line L564 (351.885, -438) -> (348.9983, -443)
  line L565 (351.885, -453) -> (348.9983, -458)
  line L566 (343.2247, -448) -> (348.9983, -448)
  line L567 (343.2247, -458) -> (340.338, -453)
  line L568 (340.338, -453) -> (343.2247, -448)
  line L569 (348.9983, -433) -> (351.885, -438)
  line L570 (348.9983, -443) -> (343.2247, -443)
  line L571 (343.2247, -443) -> (340.338, -438)
  line L572 (343.2247, -433) -> (348.9983, -433)
  line L573 (340.338, -438) -> (343.2247, -433)
  line L574 (348.9983, -428) -> (343.2247, -428)
  line L575 (351.885, -423) -> (348.9983, -428)
  line L576 (343.2247, -428) -> (340.338, -423)
  line L577 (348.9983, -418) -> (351.885, -423)
  line L578 (343.2247, -418) -> (348.9983, -418)
  line L579 (340.338, -423) -> (343.2247, -418)
  line L580 (353.3284, -430.5) -> (356.2151, -425.5)
  line L581 (356.2151, -435.5) -> (353.3284, -430.5)
  line L582 (361.9886, -435.5) -> (356.2151, -435.5)
  line L583 (364.8754, -430.5) -> (361.9886, -435.5)
  line L584 (361.9886, -425.5) -> (364.8754, -430.5)
  line L585 (356.2151, -425.5) -> (361.9886, -425.5)
  line L586 (356.2151, -420.5) -> (353.3284, -415.5)
  line L587 (353.3284, -415.5) -> (356.2151, -410.5)
  line L588 (361.9886, -420.5) -> (356.2151, -420.5)
  line L589 (356.2151, -410.5) -> (361.9886, -410.5)
  line L590 (364.8754, -415.5) -> (361.9886, -420.5)
  line L591 (361.9886, -410.5) -> (364.8754, -415.5)
  point P0 (0, 0)
  point P1 (8.1115, -453)
  point P2 (21.1019, -445.5)
  point P3 (8.1115, -438)
  point P4 (8.1115, -433)
  point P5 (8.1115, -443)
  point P6 (8.1115, -418)
  point P7 (8.1115, -423)
  point P8 (8.1115, -428)
  point P9 (21.1019, -430.5)
  point P10 (8.1115, -403)
  point P11 (8.1115, -408)
  point P12 (8.1115, -413)
  point P13 (21.1019, -415.5)
  point P14 (34.1115, -403)
  point P15 (34.1115, -408)
  point P16 (34.1115, -413)
  point P17 (47.1019, -445.5)
  point P18 (34.1115, -453)
  point P19 (34.1115, -443)
  point P20 (34.1115, -438)
  point P21 (34.1115, -433)
  point P22 (34.1115, -428)
  point P23 (34.1115, -423)
  point P24 (34.1115, -418)
  point P25 (47.1019, -430.5)
  point P26 (47.1019, -415.5)
  point P27 (60.1115, -403)
  point P28 (60.1115, -408)
  point P29 (60.1115, -413)
  point P30 (73.1019, -445.5)
  point P31 (60.1115, -453)
  point P32 (60.1115, -443)
  point P33 (60.1115, -438)
  point P34 (60.1115, -433)
  point P35 (60.1115, -428)
  point P36 (60.1115, -423)
  point P37 (60.1115, -418)
  point P38 (73.1019, -430.5)
  point P39 (73.1019, -415.5)
  point P40 (86.1115, -403)
  point P41 (86.1115, -408)
  point P42 (86.1115, -413)
  point P43 (99.1019, -445.5)
  point P44 (86.1115, -453)
  point P45 (86.1115, -443)
  point P46 (86.1115, -438)
  point P47 (86.1115, -433)
  point P48 (86.1115, -428)
  point P49 (86.1115, -423)
  point P50 (86.1115, -418)
  point P51 (99.1019, -430.5)
  point P52 (99.1019, -415.5)
  point P53 (112.1115, -403)
  point P54 (112.1115, -408)
  point P55 (112.1115, -413)
  point P56 (125.1019, -445.5)
  point P57 (112.1115, -453)
  point P58 (112.1115, -443)
  point P59 (112.1115, -438)
  point P60 (112.1115, -433)
  point P61 (112.1115, -428)
  point P62 (112.1115, -423)
  point P63 (112.1115, -418)
  point P64 (125.1019, -430.5)
  point P65 (125.1019, -415.5)
  point P66 (138.1115, -403)
  point P67 (138.1115, -408)
  point P68 (138.1115, -413)
  point P69 (151.1019, -445.5)
  point P70 (138.1115, -453)
  point P71 (138.1115, -443)
  point P72 (138.1115, -438)
  point P73 (138.1115, -433)
  point P74 (138.1115, -428)
  point P75 (138.1115, -423)
  point P76 (138.1115, -418)
  point P77 (151.1019, -430.5)
  point P78 (151.1019, -415.5)
  point P79 (164.1115, -403)
  point P80 (164.1115, -408)
  point P81 (164.1115, -413)
  point P82 (177.1019, -445.5)
  point P83 (164.1115, -453)
  point P84 (164.1115, -443)
  point P85 (164.1115, -438)
  point P86 (164.1115, -433)
  point P87 (164.1115, -428)
  point P88 (164.1115, -423)
  point P89 (164.1115, -418)
  point P90 (177.1019, -430.5)
  point P91 (177.1019, -415.5)
  point P92 (190.1115, -403)
  point P93 (190.1115, -408)
  point P94 (190.1115, -413)
  point P95 (203.1019, -445.5)
  point P96 (190.1115, -453)
  point P97 (190.1115, -443)
  point P98 (190.1115, -438)
  point P99 (190.1115, -433)
  point P100 (190.1115, -428)
  point P101 (190.1115, -423)
  point P102 (190.1115, -418)
  point P103 (203.1019, -430.5)
  point P104 (203.1019, -415.5)
  point P105 (216.1115, -403)
  point P106 (216.1115, -408)
  point P107 (216.1115, -413)
  point P108 (229.1019, -445.5)
  point P109 (216.1115, -453)
  point P110 (216.1115, -443)
  point P111 (216.1115, -438)
  point P112 (216.1115, -433)
  point P113 (216.1115, -428)
  point P114 (216.1115, -423)
  point P115 (216.1115, -418)
  point P116 (229.1019, -430.5)
  point P117 (229.1019, -415.5)
  point P118 (242.1115, -403)
  point P119 (242.1115, -408)
  point P120 (242.1115, -413)
  point P121 (255.1019, -445.5)
  point P122 (242.1115, -453)
  point P123 (242.1115, -443)
  point P124 (242.1115, -438)
  point P125 (242.1115, -433)
  point P126 (242.1115, -428)
  point P127 (242.1115, -423)
  point P128 (242.1115, -418)
  point P129 (255.1019, -430.5)
  point P130 (255.1019, -415.5)
  point P131 (268.1115, -403)
  point P132 (268.1115, -408)
  point P133 (268.1115, -413)
  point P134 (281.1019, -445.5)
  point P135 (268.1115, -453)
  point P136 (268.1115, -443)
  point P137 (268.1115, -438)
  point P138 (268.1115, -433)
  point P139 (268.1115, -428)
  point P140 (268.1115, -423)
  point P141 (268.1115, -418)
  point P142 (281.1019, -430.5)
  point P143 (281.1019, -415.5)
  point P144 (294.1115, -403)
  point P145 (294.1115, -408)
  point P146 (294.1115, -413)
  point P147 (307.1019, -445.5)
  point P148 (294.1115, -453)
  point P149 (294.1115, -443)
  point P150 (294.1115, -438)
  point P151 (294.1115, -433)
  point P152 (294.1115, -428)
  point P153 (294.1115, -423)
  point P154 (294.1115, -418)
  point P155 (307.1019, -430.5)
  point P156 (307.1019, -415.5)
  point P157 (320.1115, -403)
  point P158 (320.1115, -408)
  point P159 (320.1115, -413)
  point P160 (333.1019, -445.5)
  point P161 (320.1115, -453)
  point P162 (320.1115, -443)
  point P163 (320.1115, -438)
  point P164 (320.1115, -433)
  point P165 (320.1115, -428)
  point P166 (320.1115, -423)
  point P167 (320.1115, -418)
  point P168 (333.1019, -430.5)
  point P169 (333.1019, -415.5)
  point P170 (346.1115, -403)
  point P171 (346.1115, -408)
  point P172 (346.1115, -413)
  point P173 (359.1019, -445.5)
  point P174 (346.1115, -453)
  point P175 (346.1115, -443)
  point P176 (346.1115, -438)
  point P177 (346.1115, -433)
  point P178 (346.1115, -428)
  point P179 (346.1115, -423)
  point P180 (346.1115, -418)
  point P181 (359.1019, -430.5)
  point P182 (359.1019, -415.5)
  dimension "d39" = 5
  dimension "d40" = 5
  dimension "d41" = 5
  dimension "d42" = 10
  dimension "d43" = 22
  dimension "d44" = 23.1115
  dimension "d47" = 15
  dimension "d63" = 26
  constraints: 1176 end point, 4 horizontal, 2 equal length, 2 midpoint, 1 vertical, 1 vertical alignment, 1356 other
  measures "d39" distance between parallel lines of L8 L10
  measures "d40" distance between parallel lines of L11 L21
  measures "d41" distance between parallel lines of L7 L16
  measures "d42" distance of point (8.111, -433) point (8.111, -443)
  measures "d43" distance between parallel lines of L0 L4
  measures "d44" distance from line of L3 point (8.111, -453)
  measures "d47" distance of point (8.111, -433) point (8.111, -418)
  measures "d63" distance of L34.end L46.start
extrude "Extrusion3" cut sketch "Sketch4" against normal through all contours L4 L5 L6 L7 L8 L9 | L10 L11 L12 L13 L14 L15 | L16 L17 L18 L19 L20 L21 | L22 L24 L28 L27 L26 L23 | L25 L30 L33 L32 L31 L29 | L34 L36 L40 L39 L38 L35 | L37 L42 L45 L44 L43 L41 | L46 L48 L51 L50 L49 L47 | L52 L53 L54 L55 L57 L56 | L58 L63 L64 L62 L59 L61 | L60 L66 L67 L69 L68 L65 | L70 L72 L75 L74 L73 L71 | L76 L81 L80 L79 L78 L77 | L82 L83 L85 L87 L86 L84 | L88 L90 L93 L92 L91 L89 | L94 L95 L96 L97 L99 L98 | L100 L105 L106 L104 L101 L103 | L102 L108 L109 L111 L110 L107 | L112 L114 L117 L116 L115 L113 | L118 L123 L122 L121 L120 L119 | L124 L125 L127 L129 L128 L126 | L130 L132 L135 L134 L133 L131 | L136 L137 L138 L139 L141 L140 | L142 L147 L148 L146 L143 L145 | L144 L150 L151 L153 L152 L149 | L154 L156 L159 L158 L157 L155 | L160 L165 L164 L163 L162 L161 | L166 L167 L169 L171 L170 L168 | L172 L174 L177 L176 L175 L173 | L178 L179 L180 L181 L183 L182 | L184 L189 L190 L188 L185 L187 | L186 L192 L193 L195 L194 L191 | L196 L198 L201 L200 L199 L197 | L202 L207 L206 L205 L204 L203 | L208 L209 L211 L213 L212 L210 | L214 L216 L219 L218 L217 L215 | L220 L221 L222 L223 L225 L224 | L226 L231 L232 L230 L227 L229 | L228 L234 L235 L237 L236 L233 | L238 L240 L243 L242 L241 L239 | L244 L249 L248 L247 L246 L245 | L250 L251 L253 L255 L254 L252 | L256 L258 L261 L260 L259 L257 | L262 L263 L264 L265 L267 L266 | L268 L273 L274 L272 L269 L271 | L270 L276 L277 L279 L278 L275 | L280 L282 L285 L284 L283 L281 | L286 L291 L290 L289 L288 L287 | L292 L293 L295 L297 L296 L294 | L298 L300 L303 L302 L301 L299 | L304 L305 L306 L307 L309 L308 | L310 L315 L316 L314 L311 L313 | L312 L318 L319 L321 L320 L317 | L322 L324 L327 L326 L325 L323 | L328 L333 L332 L331 L330 L329 | L334 L335 L337 L339 L338 L336 | L340 L342 L345 L344 L343 L341 | L346 L347 L348 L349 L351 L350 | L352 L357 L358 L356 L353 L355 | L354 L360 L361 L363 L362 L359 | L364 L366 L369 L368 L367 L365 | L370 L375 L374 L373 L372 L371 | L376 L377 L379 L381 L380 L378 | L382 L384 L387 L386 L385 L383 | L388 L389 L390 L391 L393 L392 | L394 L399 L400 L398 L395 L397 | L396 L402 L403 L405 L404 L401 | L406 L408 L411 L410 L409 L407 | L412 L417 L416 L415 L414 L413 | L418 L419 L421 L423 L422 L420 | L424 L426 L429 L428 L427 L425 | L430 L431 L432 L433 L435 L434 | L436 L441 L442 L440 L437 L439 | L438 L444 L445 L447 L446 L443 | L448 L450 L453 L452 L451 L449 | L454 L459 L458 L457 L456 L455 | L460 L461 L463 L465 L464 L462 | L466 L468 L471 L470 L469 L467 | L472 L473 L474 L475 L477 L476 | L478 L483 L484 L482 L479 L481 | L480 L486 L487 L489 L488 L485 | L490 L492 L495 L494 L493 L491 | L496 L501 L500 L499 L498 L497 | L502 L503 L505 L507 L506 L504 | L508 L510 L513 L512 L511 L509 | L514 L515 L516 L517 L519 L518 | L520 L525 L526 L524 L521 L523 | L522 L528 L529 L531 L530 L527 | L532 L534 L537 L536 L535 L533 | L538 L543 L542 L541 L540 L539 | L544 L545 L547 L549 L548 L546 | L550 L552 L555 L554 L553 L551 | L562 L567 L568 L566 L563 L565 | L564 L570 L571 L573 L572 L569 | L574 L576 L579 L578 L577 L575